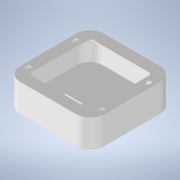
# Autodesk Inventor part: housing_new
Saved by Autodesk Inventor 2021 (Build 250183000, 183)
## iProperties
Created: 2020-09-29
Part Number: housing_new
Material: Generisch
Document SubType Name: Modeling
Designer: Ben
Density: 1 g/cm^3
Appearance: Vorgabe
Author: Ben
Autodesk Inventor part; units mm, degrees
note: some values were not read from the file. Chosen so that the rebuilt part matches the saved one: direction of "Bohrung1"; direction of "Bohrung2"; direction of "Bohrung3"; direction of "Bohrung4".
sketch "Skizze1" plane through (0, 0, 0) normal (0, 1, 0) x (-1, 0, 0)
  line L0 (10, 0) -> (50, 0)
  line L1 (60, -10) -> (60, -50)
  line L2 (50, -60) -> (10, -60)
  line L3 (0, -50) -> (0, -10)
  arc A0 (60, -10) -> (50, 0) centre (50, -10) ccw
  arc A1 (50, -60) -> (60, -50) centre (50, -50) ccw
  arc A2 (0, -50) -> (10, -60) centre (10, -50) ccw
  arc A3 (10, 0) -> (0, -10) centre (10, -10) ccw
  point P0 (0, 0)
  point P1 (60, -60)
  point P2 (60, 0)
  point P3 (0, -60)
  dimension "d0" = 60
  dimension "d1" = 60
  dimension "d2" = 10
  constraints: 8 end point, 8 point on circle, 8 point on line, 8 tangent, 4 centre point, 3 equal radius, 2 parallel, 1 horizontal, 1 perpendicular
  measures "d0" distance of point (60, 0) point (60, -60)
  measures "d1" distance of point (60, -60) point (0, -60)
  measures "d2" radius of A0
extrude "Extrusion1" add sketch "Skizze1" along normal blind 1
sketch "Skizze4" plane through (0, 1, 0) normal (0, 1, 0) x (1, 0, 0)
  line L0 (-10, 60) -> (-50, 60) projected
  arc A0 (-50, 60) -> (-60, 50) centre (-50, 50) ccw projected
  line L1 (-60, 50) -> (-60, 10) projected
  arc A1 (-60, 10) -> (-50, 0) centre (-50, 10) ccw projected
  line L2 (-50, 0) -> (-10, 0) projected
  arc A2 (-10, 0) -> (0, 10) centre (-10, 10) ccw projected
  line L3 (0, 10) -> (0, 50) projected
  arc A3 (0, 50) -> (-10, 60) centre (-10, 50) ccw projected
  arc A4 (-10, 1) -> (-1, 10) centre (-10, 10) ccw
  line L4 (-10, 1) -> (-50, 1)
  arc A5 (-59, 10) -> (-50, 1) centre (-50, 10) ccw
  line L5 (-59, 10) -> (-59, 50)
  arc A6 (-50, 59) -> (-59, 50) centre (-50, 50) ccw
  line L6 (-50, 59) -> (-10, 59)
  arc A7 (-1, 50) -> (-10, 59) centre (-10, 50) ccw
  line L7 (-1, 50) -> (-1, 10)
  arc A8 (-10, 0) -> (0, 10) centre (-10, 10) ccw
  line L8 (-10, 0) -> (-50, 0)
  arc A9 (-60, 10) -> (-50, 0) centre (-50, 10) ccw
  line L9 (-60, 10) -> (-60, 50)
  arc A10 (-50, 60) -> (-60, 50) centre (-50, 50) ccw
  line L10 (-50, 60) -> (-10, 60)
  arc A11 (0, 50) -> (-10, 60) centre (-10, 50) ccw
  line L11 (0, 50) -> (0, 10)
  dimension "d7" = 1
  dimension "d8" = 1
  constraints: 16 end point, 16 point on circle, 8 centre point, 14 other
  measures "d7" radial gap between concentric circles of A2 A4
  measures "d8" radial gap between concentric circles of A4 A8
extrude "Extrusion2" add sketch "Skizze4" along normal blind 18
sketch "Skizze5" plane through (0, 19, 0) normal (0, 1, 0) x (1, 0, 0)
  arc A0 (-10, 0) -> (0, 10) centre (-10, 10) ccw projected
  line L0 (0, 10) -> (0, 50) projected
  arc A1 (0, 50) -> (-10, 60) centre (-10, 50) ccw projected
  line L1 (-10, 60) -> (-50, 60) projected
  arc A2 (-50, 60) -> (-60, 50) centre (-50, 50) ccw projected
  line L2 (-60, 50) -> (-60, 10) projected
  arc A3 (-60, 10) -> (-50, 0) centre (-50, 10) ccw projected
  line L3 (-50, 0) -> (-10, 0) projected
  arc A4 (-10, 8) -> (-8, 10) centre (-10, 10) ccw
  line L4 (-10, 8) -> (-50, 8)
  arc A5 (-52, 10) -> (-50, 8) centre (-50, 10) ccw
  line L5 (-52, 10) -> (-52, 50)
  arc A6 (-50, 52) -> (-52, 50) centre (-50, 50) ccw
  line L6 (-50, 52) -> (-10, 52)
  arc A7 (-8, 50) -> (-10, 52) centre (-10, 50) ccw
  line L7 (-8, 50) -> (-8, 10)
  line L8 (-50, 0) -> (-10, 0)
  arc A8 (-10, 0) -> (0, 10) centre (-10, 10) ccw
  line L9 (0, 10) -> (0, 50)
  arc A9 (0, 50) -> (-10, 60) centre (-10, 50) ccw
  line L10 (-10, 60) -> (-50, 60)
  arc A10 (-50, 60) -> (-60, 50) centre (-50, 50) ccw
  line L11 (-60, 50) -> (-60, 10)
  arc A11 (-60, 10) -> (-50, 0) centre (-50, 10) ccw
  point P0 (0, 0)
  dimension "d11" = 8
  dimension "d12" = 8
  constraints: 16 end point, 16 point on circle, 8 centre point, 14 other
  measures "d11" radial gap between concentric circles of A0 A4
  measures "d12" distance between parallel lines of L4 L8
extrude "Extrusion3" add sketch "Skizze5" along normal blind 1
fillet "Rundung1" radius 0.2 48 edges at (-57.0711, 0, -57.0711) (-60, 0, -30) (-57.0711, 0, -2.9289) (-30, 0, 0) (-2.9289, 0, -2.9289) (0, 0, -30) (-2.9289, 0, -57.0711) (-30, 0, -60) (-1, 1, -30) (-3.636, 1, -56.364) (-30, 1, -59) (-56.364, 1, -56.364) (-59, 1, -30) (-56.364, 1, -3.636) (-30, 1, -1) (-3.636, 1, -3.636) (-51.4142, 19, -8.5858) (-52, 19, -30) (-51.4142, 19, -51.4142) (-30, 19, -52) (-8.5858, 19, -51.4142) (-8, 19, -30) (-8.5858, 19, -8.5858) (-30, 19, -8) (-56.364, 19, -3.636) (-59, 19, -30) (-56.364, 19, -56.364) (-30, 19, -59) (-3.636, 19, -56.364) (-1, 19, -30) (-3.636, 19, -3.636) (-30, 19, -1) (-57.0711, 20, -2.9289) (-30, 20, 0) (-2.9289, 20, -2.9289) (0, 20, -30) (-2.9289, 20, -57.0711) (-30, 20, -60) (-57.0711, 20, -57.0711) (-60, 20, -30) (-8.5858, 20, -51.4142) (-8, 20, -30) (-8.5858, 20, -8.5858) (-30, 20, -8) (-51.4142, 20, -8.5858) (-52, 20, -30) (-51.4142, 20, -51.4142) (-30, 20, -52)
sketch "Skizze6" plane through (0, 20, 0) normal (0, 1, 0) x (1, 0, 0)
  line L0 (-7.8, 10) -> (-7.8, 50) projected
  line L1 (-52.2, 50) -> (-52.2, 10) projected
  line L2 (-10, 0.2) -> (-50, 0.2) projected
  line L3 (-3.8, 12.2) -> (-3.8, 45.8)
  line L4 (-56.2, 12.2) -> (-56.2, 45.8)
  line L5 (-3.8, 45.8) -> (-56.2, 45.8)
  line L6 (-10, 52.2) -> (-50, 52.2) projected
  line L7 (-50, 59.8) -> (-10, 59.8) projected
  line L8 (-3.8, 12.2) -> (-56.2, 12.2)
  line L9 (-50, 7.8) -> (-10, 7.8) projected
  point P0 (0, 0)
  dimension "d23" = 4
  dimension "d24" = 4
  dimension "d25" = 12
  dimension "d26" = 14
  constraints: 8 end point, 4 parallel
  measures "d23" distance from line of L0 L3.start
  measures "d24" distance from line of L4.start L1
  measures "d25" distance from line of L3.start L2
  measures "d26" distance between parallel lines of L7 L5
hole "Bohrung1" at (-3.8, 20, -12.2) at (-3.8, 20, -45.8) at (-56.2, 20, -12.2) at (-56.2, 20, -45.8) direction (0, -1, 0) diameter 3 depth 1
sketch "Skizze7" plane through (0, 20, 0) normal (0, 1, 0) x (1, 0, 0)
  circle A0 centre (-3.8, 12.2) radius 1.5 projected
  circle A1 centre (-3.8, 45.8) radius 1.5 projected
  circle A2 centre (-56.2, 45.8) radius 1.5 projected
  circle A3 centre (-56.2, 12.2) radius 1.5 projected
  line L0 (-3.8, 10.7) -> (-3.8, 44.3)
  line L1 (-56.2, 10.7) -> (-56.2, 44.3)
  point P0 (0, 0)
  constraints: 4 end point, 4 vertical alignment, 2 point on line, 2 vertical, 4 other
hole "Bohrung2" at (-3.8, 20, -10.7) at (-3.8, 20, -44.3) at (-56.2, 20, -44.3) at (-56.2, 20, -10.7) direction (0, -1, 0) diameter 2 depth 1
sketch "Skizze8" plane through (0, 1, 0) normal (0, 1, 0) x (1, 0, 0)
  circle A0 centre (-39.0725, 21.3988) radius 1.6 projected
  line L0 (-43.2, 25.3675) -> (-16.2125, 25.3675) projected
  line L1 (-43.2, 6) -> (-43.2, 25.3675) projected
  line L2 (-16.2125, 6) -> (-43.2, 6) projected
  line L3 (-43.7, 25.8675) -> (-43.7, 5.5)
  line L4 (-43.7, 5.5) -> (-16.2125, 5.5)
  line L5 (-43.2, 25.3675) -> (-43.2, 6)
  line L6 (-43.2, 6) -> (-16.2125, 6)
  line L7 (-16.2125, 25.8675) -> (-16.2125, 25.3675)
  line L8 (-16.2125, 6) -> (-16.2125, 5.5)
  line L9 (-30.0237, 25.05) -> (-30.0237, 19.97) projected
  line L10 (-24.15, 19.97) -> (-24.15, 25.05) projected
  line L11 (-31.0237, 25.8675) -> (-31.0237, 25.3675)
  line L12 (-23.15, 25.8675) -> (-23.15, 25.3675)
  line L13 (-16.2125, 25.8675) -> (-23.15, 25.8675)
  line L14 (-31.0237, 25.8675) -> (-43.7, 25.8675)
  line L15 (-16.2125, 25.3675) -> (-23.15, 25.3675)
  line L16 (-31.0237, 25.3675) -> (-43.2, 25.3675)
  line L17 (-40.5515, 21.1488) -> (-37.5935, 21.1488)
  line L18 (-37.5935, 21.6488) -> (-40.5515, 21.6488)
  arc A1 (-37.5935, 21.6488) -> (-40.5515, 21.6488) centre (-39.0725, 21.3988) ccw
  arc A2 (-40.5515, 21.1488) -> (-37.5935, 21.1488) centre (-39.0725, 21.3988) ccw
  point P0 (0, 0)
  dimension "d35" = 0.5
  dimension "d37" = 27.4875
  dimension "d38" = 27.4875
  dimension "d39" = 1
  dimension "d40" = 1
  dimension "d41" = 0.5
  dimension "d42" = 0.5
  dimension "d44" = 13.1763
  dimension "d62" = 0.5
  dimension "d63" = 1.5
  dimension "d64" = 1.5
  dimension "d65" = 2.958
  constraints: 28 end point, 4 perpendicular, 4 point on circle, 2 centre point, 2 collinear, 2 equal length, 1 horizontal, 2 other
  measures "d35" distance between parallel lines of L1 L3
  measures "d37" distance between parallel lines of L3 L7
  measures "d38" distance between parallel lines of L3 L8
  measures "d39" distance between parallel lines of L11 L9
  measures "d40" distance between parallel lines of L12 L10
  measures "d41" distance between parallel lines of L0 L13
  measures "d42" distance between parallel lines of L0 L14
  measures "d44" distance between parallel lines of L9 L5
  measures "d62" distance between parallel lines of L18 L17
  measures "d63" radius of A2
  measures "d64" radius of A1
  measures "d65" distance of L17.start L17.end
ref_plane "Arbeitsebene1" through (-43.2, 3.55, -25.3675) normal (0, 1, 0) x (0, 0, 1)
extrude "Extrusion4" add sketch "Skizze8" along normal up to surface (2.55 mm away) contours L1 L2 L8 L4 L3 L14 L11 L0 | L12 L13 L7 L0 | L17 A2 | L18 A1
sketch "Skizze9" plane through (0, 1, 0) normal (0, 1, 0) x (1, 0, 0)
  line L0 (-34.2, 22.3675) -> (-33.2, 22.3675)
  line L1 (-33.2, 22.3675) -> (-33.2, 10.3675)
  line L2 (-33.2, 10.3675) -> (-34.2, 10.3675)
  line L3 (-34.2, 10.3675) -> (-34.2, 22.3675)
  line L4 (-41.2, 17.3675) -> (-34.2, 17.3675)
  line L5 (-34.2, 17.3675) -> (-34.2, 16.3675)
  line L6 (-34.2, 16.3675) -> (-41.2, 16.3675)
  line L7 (-41.2, 16.3675) -> (-41.2, 17.3675)
  line L8 (-36.2, 10.3675) -> (-19.2, 10.3675)
  line L9 (-19.2, 10.3675) -> (-19.2, 9.3675)
  line L10 (-19.2, 9.3675) -> (-36.2, 9.3675)
  line L11 (-36.2, 9.3675) -> (-36.2, 10.3675)
  line L12 (-33.2, 19.2221) -> (-25.2, 19.2221)
  line L13 (-25.2, 19.2221) -> (-25.2, 18.2221)
  line L14 (-25.2, 18.2221) -> (-33.2, 18.2221)
  line L15 (-33.2, 18.2221) -> (-33.2, 19.2221)
  line L16 (-43.2, 25.3675) -> (-16.2125, 25.3675) projected
  line L17 (-43.2, 6) -> (-43.2, 25.3675) projected
  point P0 (0, 0)
  dimension "d47" = 1
  dimension "d48" = 12
  dimension "d49" = 3
  dimension "d50" = 1
  dimension "d51" = 17
  dimension "d52" = 7
  dimension "d53" = 1
  dimension "d54" = 7
  dimension "d55" = 2
  dimension "d56" = 8
  dimension "d57" = 1
  dimension "d58" = 3.1454
  constraints: 32 end point, 8 parallel, 4 horizontal, 4 perpendicular, 2 point on line, 1 midpoint
  measures "d47" distance of L1.end L2.end
  measures "d48" distance of L2.end L0.start
  measures "d49" distance between parallel lines of L16 L0
  measures "d50" distance of L8.end L9.end
  measures "d51" distance of L9.end L10.end
  measures "d52" distance between parallel lines of L17 L11
  measures "d53" distance of L6.end L4.start
  measures "d54" distance of L4.start L4.end
  measures "d55" distance between parallel lines of L17 L7
  measures "d56" distance of L13.end L14.end
  measures "d57" distance between parallel lines of L14 L12
  measures "d58" distance between parallel lines of L0 L12
ref_plane "Arbeitsebene2" through (-43.2, 3.55, -25.3675) normal (0, 1, 0) x (0, 0, 1)
ref_plane "Arbeitsebene3" through (-43.2, 2, -25.3675) normal (0, -1, 0) x (1, 0, 0)
extrude "Extrusion5" add sketch "Skizze9" along normal up to surface (1 mm away)
sketch "Skizze10" plane through (-39.0725, 3.55, -21.3988) normal (0, 1, 0) x (1, 0, 0)
  arc A0 (-1.479, -0.25) -> (1.479, -0.25) centre (0, 0) ccw projected
  line L0 (-1.479, -0.25) -> (1.479, -0.25) projected
  line L1 (1.479, 0.25) -> (-1.479, 0.25) projected
  arc A1 (1.479, 0.25) -> (-1.479, 0.25) centre (0, 0) ccw projected
  point P0 (39.0725, -21.3988)
extrude "Extrusion6" add sketch "Skizze10" along normal blind 0.2
ref_plane "Arbeitsebene4" through (-37.5935, 3.55, -21.1488) normal (-1, 0, 0) x (0, 1, 0)
sketch "Skizze11" plane through (-37.5935, 3.55, -21.1488) normal (-1, 0, 0) x (0, 1, 0)
  line L0 (-2.55, 0) -> (0.2, 0) projected
  line L1 (-2.55, 0.5) -> (0.2, 0.5) projected
  line L2 (-2.55, 0) -> (-2.55, -1.25) projected
  line L3 (-2.55, 1.75) -> (-2.55, 0.5) projected
  line L4 (0.2, 0.5) -> (0.2, 1.75) projected
  line L5 (0.2, -1.25) -> (0.2, 0) projected
  line L6 (0.2, -1.25) -> (-2.55, -1.25)
  line L7 (-2.55, -1.25) -> (-2.55, 1.75)
  line L8 (-2.55, 1.75) -> (0.2, 1.75)
  line L9 (0.2, 1.75) -> (0.2, -1.25)
  point P0 (-3.55, -21.1488)
  constraints: 8 end point, 2 parallel, 1 horizontal, 1 perpendicular
extrude "Extrusion7" cut sketch "Skizze11" along normal blind 0.3
ref_plane "Arbeitsebene5" through (-40.5515, 3.55, -21.6488) normal (1, 0, 0) x (0, 1, 0)
sketch "Skizze12" plane through (-40.5515, 3.55, -21.6488) normal (1, 0, 0) x (0, 1, 0)
  line L0 (-2.55, 1.75) -> (0.2, 1.75) projected
  line L1 (-2.55, -1.25) -> (0.2, -1.25) projected
  line L2 (-2.55, 0) -> (-2.55, -1.25) projected
  line L3 (-2.55, 1.75) -> (-2.55, 0.5) projected
  line L4 (0.2, -1.25) -> (0.2, 0) projected
  line L5 (0.2, 0.5) -> (0.2, 1.75) projected
  line L6 (0.2, -1.25) -> (-2.55, -1.25)
  line L7 (-2.55, -1.25) -> (-2.55, 1.75)
  line L8 (-2.55, 1.75) -> (0.2, 1.75)
  line L9 (0.2, 1.75) -> (0.2, -1.25)
  point P0 (-3.55, 21.6488)
  point P1 (-2.55, -0.6773)
  point P2 (-2.55, 1.1773)
  point P3 (0.2, -0.6773)
  point P4 (0.2, 1.1773)
  constraints: 8 end point, 2 parallel, 1 horizontal, 1 perpendicular
extrude "Extrusion8" cut sketch "Skizze12" along normal blind 0.3
sketch "Skizze13" plane through (-39.0725, 3.75, -21.3988) normal (0, 1, 0) x (1, 0, 0)
  line L0 (-1.179, 0.9273) -> (-1.179, 0.25) projected
  line L1 (-1.179, 0.25) -> (1.179, 0.25) projected
  line L2 (1.179, 0.25) -> (1.179, 0.9273) projected
  arc A0 (1.179, 0.9273) -> (-1.179, 0.9273) centre (0, 0) ccw projected
  line L3 (-1.179, -0.25) -> (-1.179, -0.9273) projected
  arc A1 (-1.179, -0.9273) -> (1.179, -0.9273) centre (0, 0) ccw projected
  line L4 (1.179, -0.9273) -> (1.179, -0.25) projected
  line L5 (1.179, -0.25) -> (-1.179, -0.25) projected
  arc A2 (1.179, 1.2247) -> (-1.179, 1.2247) centre (0, 0) ccw
  line L6 (1.179, 0.9273) -> (1.179, 0.25) projected
  line L7 (1.179, 0.25) -> (-1.179, 0.25) projected
  arc A3 (1.179, 0.9273) -> (-1.179, 0.9273) centre (0, 0) ccw projected
  line L8 (1.179, 0.9273) -> (1.179, 1.2247)
  line L9 (-1.179, 0.9273) -> (-1.179, 1.2247)
  arc A4 (-1.179, -1.2247) -> (1.179, -1.2247) centre (0, 0) ccw
  line L10 (1.179, -0.25) -> (1.179, -0.9273) projected
  line L11 (1.179, -0.9273) -> (1.179, -1.2247)
  arc A5 (-1.179, -0.9273) -> (1.179, -0.9273) centre (0, 0) ccw projected
  line L12 (-1.179, -0.9273) -> (-1.179, -1.2247)
  line L13 (1.179, 0.9273) -> (1.179, 0.25)
  line L14 (-1.179, 0.25) -> (-1.179, 0.9273) projected
  line L15 (-1.179, 0.25) -> (-1.179, 0.9273)
  line L16 (1.179, -0.9273) -> (1.179, -0.25)
  line L17 (1.179, -0.25) -> (-1.179, -0.25) projected
  line L18 (-1.179, -0.25) -> (-1.179, -0.9273) projected
  line L19 (-1.179, -0.25) -> (-1.179, -0.9273)
  point P0 (39.0725, -21.3988)
  dimension "d72" = 0.2
  dimension "d73" = 0.2
  constraints: 16 end point, 5 equal length, 4 point on circle, 2 centre point, 2 point on line, 1 vertical
  measures "d72" radial gap between concentric circles of A0 A2
  measures "d73" radial gap between concentric circles of A1 A4
extrude "Extrusion9" add sketch "Skizze13" along normal blind 1.5
chamfer "Fase1" distance 1.2 angle 45 2 edges at (-39.0725, 5.25, -23.0988) (-39.0725, 5.25, -19.6988)
sketch "Skizze14" plane through (0, 0, 0) normal (0, -1, 0) x (1, 0, 0)
  point P0 (0, 0)
  point P1 (-18.0895, -16.1224)
hole "Bohrung3" at (-18.0895, 0, -16.1224) direction (0, 1, 0) diameter 2 depth 1
sketch "Skizze15" plane through (0, 0, 0) normal (0, -1, 0) x (1, 0, 0)
  point P0 (0, 0)
  point P1 (-40.5049, -10.6572)
hole "Bohrung4" at (-40.5049, 0, -10.6572) direction (0, 1, 0) diameter 1.5 depth 1
chamfer "Fase2" distance 1 angle 45 1 edges at (-18.0895, 0, -15.1224)
